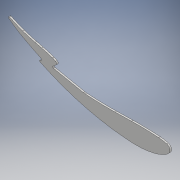
# Autodesk Inventor part: bracket1
Saved by Autodesk Inventor 2018.2 (Build 222227000, 227)
## iProperties
Created: 2018-03-05
Part Number: bracket1
Material: 一般
Document SubType Name: Modeling
Designer: ku_sk
Density: 1 g/cm^3
Appearance: 既定
Author: ku_sk
Autodesk Inventor part; units mm, degrees
ref_plane "YZ Plane" through (0, 0, 0) normal (1, 0, 0) x (0, 1, 0)
ref_plane "XZ Plane" through (0, 0, 0) normal (0, 1, 0) x (-1, 0, 0)
ref_plane "XY Plane" through (0, 0, 0) normal (0, 0, 1) x (1, 0, 0)
sketch "スケッチ1" plane through (0, 0, 0) normal (0, 1, 0) x (-1, 0, 0)
  arc A0 (73.3541, 27.446) -> (-100.3009, 51.217) centre (-120.0382, -739.1608) ccw projected
  arc A1 (-35.9382, 7.5619) -> (73.3541, 27.446) centre (-88.8837, 608.8772) ccw projected
  arc A2 (-61.641, 6.0637) -> (-35.9382, 7.5619) centre (-74.0904, 440.8658) ccw projected
  arc A3 (-109.3953, 11.1574) -> (-61.641, 6.0637) centre (-66.7514, 184.549) ccw projected
  arc A4 (-137.5577, 22.6319) -> (-109.3953, 11.1574) centre (-84.3921, 112.8213) ccw projected
  arc A5 (-145.8114, 29.5987) -> (-137.5577, 22.6319) centre (-121.1943, 50.3906) ccw projected
  arc A6 (-140.2753, 46.8162) -> (-145.8114, 29.5987) centre (-137.666, 36.4784) ccw projected
  arc A7 (-120.2839, 50.0437) -> (-140.2753, 46.8162) centre (-111.8153, -65.9388) ccw projected
  arc A8 (-100.3009, 51.217) -> (-120.2839, 50.0437) centre (-69.1096, -650.8128) ccw projected
  arc A9 (174.7503, 65.8482) -> (173.4237, 69.5954) centre (173.8768, 67.6474) ccw projected
  arc A10 (64.7746, 52.985) -> (173.4237, 69.5954) centre (11.2401, 766.801) ccw projected
  arc A11 (-11.9173, 50.8598) -> (64.7746, 52.985) centre (3.9096, 864.5436) ccw projected
  arc A12 (-53.1769, 51.7289) -> (-11.9173, 50.8598) centre (236.8377, 12839.6895) ccw projected
  arc A13 (-53.1769, 51.7289) -> (-120.2839, 50.0437) centre (-69.1096, -650.8128) ccw projected
  arc A14 (-120.2839, 50.0437) -> (-140.2753, 46.8162) centre (-111.8153, -65.9388) ccw projected
  arc A15 (-140.2753, 46.8162) -> (-145.8114, 29.5987) centre (-137.666, 36.4784) ccw projected
  arc A16 (-145.8114, 29.5987) -> (-137.5577, 22.6319) centre (-121.1943, 50.3906) ccw projected
  arc A17 (-137.5577, 22.6319) -> (-109.3953, 11.1574) centre (-84.3921, 112.8213) ccw projected
  arc A18 (-109.3953, 11.1574) -> (-61.641, 6.0637) centre (-66.7514, 184.549) ccw projected
  arc A19 (-61.641, 6.0637) -> (-35.9382, 7.5619) centre (-74.0904, 440.8658) ccw projected
  arc A20 (-35.9382, 7.5619) -> (174.7503, 65.8482) centre (-88.8837, 608.8772) ccw projected
  arc A21 (252.3508, 120.9538) -> (250.2273, 124.316) centre (251.1064, 122.5195) ccw projected
  arc A22 (217.6526, 110.7016) -> (250.2273, 124.316) centre (119.1278, 392.2173) ccw projected
  arc A23 (187.0157, 101.5757) -> (217.6526, 110.7016) centre (105.6368, 430.7651) ccw projected
  arc A24 (170.3162, 97.476) -> (187.0157, 101.5757) centre (-1092.0317, 5275.5105) ccw projected
  arc A25 (170.3162, 97.476) -> (143.4895, 89.5609) centre (239.6668, -186.9935) ccw projected
  arc A26 (143.4895, 89.5609) -> (135.7916, 86.106) centre (159.4055, 43.7948) ccw projected
  arc A27 (135.7916, 86.106) -> (135.4203, 78.5795) centre (137.9566, 82.2268) ccw projected
  arc A28 (135.4203, 78.5795) -> (139.4934, 76.6657) centre (143.0857, 89.6023) ccw projected
  arc A29 (139.4934, 76.6657) -> (152.0654, 75.0846) centre (151.1648, 118.6976) ccw projected
  arc A30 (152.0654, 75.0846) -> (171.8343, 78.1844) centre (150.5294, 149.4681) ccw projected
  arc A31 (171.8343, 78.1844) -> (182.0173, 81.5592) centre (119.9342, 251.8363) ccw projected
  arc A32 (182.0173, 81.5592) -> (252.3508, 120.9538) centre (95.8618, 317.8604) ccw projected
  line L0 (209.5049, 93.4807) -> (167.3677, 72.1392)
  line L1 (167.3677, 72.1392) -> (174.5596, 69.5273)
  line L2 (135.0309, 78.8838) -> (145.7217, 69.5273)
  line L3 (145.7217, 69.5273) -> (64.7746, 52.985)
  point P0 (0, 0)
  constraints: 8 end point, 3 point on circle, 3 tangent
extrude "押し出し1" add sketch "スケッチ1" along normal blind 4
fillet "フィレット1" radius 2 1 edges at (-145.7217, 2, 69.5273)
fillet "フィレット1" radius 30 1 edges at (-64.7746, 2, 52.985)
fillet "フィレット1" radius 2 1 edges at (-167.3677, 2, 72.1392)
